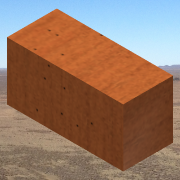
# Autodesk Inventor part: endWoodblock
Saved by Autodesk Inventor 2014 SP1 (Build 180222100, 222)
## iProperties
Created: 2014-05-19
Part Number: endWoodblock
Material: Wood (Cherry)
Document SubType Name: Modeling
Designer: Dave
Mass: 94.8504 g
Surface Area: 180.645 cm^2
Volume: 150.556 cm^3
Density: 0.63 g/cm^3
Appearance: Cherry - Natural Low Gloss
Author: Dave
Autodesk Inventor part; units mm, degrees
ref_plane "YZ Plane" through (0, 0, 0) normal (1, 0, 0) x (0, 1, 0)
ref_plane "XZ Plane" through (0, 0, 0) normal (0, 1, 0) x (-1, 0, 0)
ref_plane "XY Plane" through (0, 0, 0) normal (0, 0, 1) x (1, 0, 0)
sketch "Sketch1" plane through (0, 0, 0) normal (0, 0, 1) x (1, 0, 0)
  line L0 (0, 0) -> (88.9, 0)
  line L1 (88.9, 0) -> (88.9, 44.45)
  line L2 (88.9, 44.45) -> (0, 44.45)
  line L3 (0, 44.45) -> (0, 0)
  dimension "d0" = 88.9
  dimension "d1" = 44.45
  constraints: 8 end point, 2 parallel, 1 horizontal, 1 perpendicular
  measures "d0" distance of L2.end L1.end
  measures "d1" distance of L1.end L0.end
extrude "Extrusion1" add sketch "Sketch1" along normal blind 38.1
body "Solid1"
